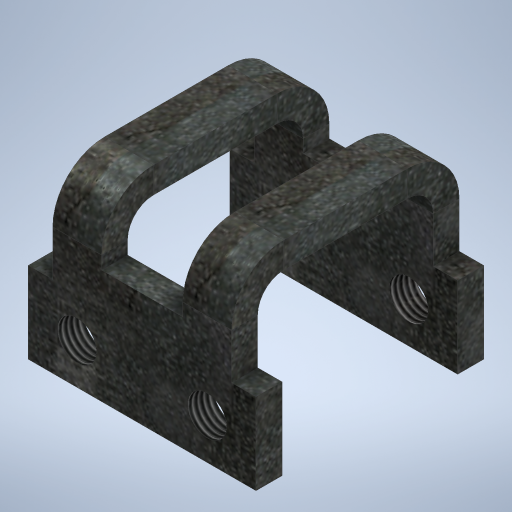
# Autodesk Inventor part: Encaixe Macaco
Saved by Autodesk Inventor 2024 (Build 280153000, 153)
## iProperties
Created: 2024-06-03
Part Number: Encaixe Macaco
Material: Steel ASTM A36
Document SubType Name: Sheet Metal
Designer: Pedro
Density: 7.85 g/cm^3
Sheet Metal Rule: Default_mm
Appearance: Plate
Mass: 418.159 g
Surface Area: 200.819 cm^2
Volume: 53.2687 cm^3
Author: Pedro
Autodesk Inventor part; units mm, degrees
ref_plane "YZ Plane" through (0, 0, 0) normal (1, 0, 0) x (0, 1, 0)
ref_plane "XZ Plane" through (0, 0, 0) normal (0, 1, 0) x (-1, 0, 0)
ref_plane "XY Plane" through (0, 0, 0) normal (0, 0, 1) x (1, 0, 0)
sketch "Sketch1" plane through (0, 0, 0) normal (0, 0, 1) x (1, 0, 0)
  line L0 (2.0005, 12.9652) -> (57.0005, 12.9652)
  line L1 (17.0005, -7.0348) -> (17.0005, 12.9652)
  line L2 (42.0005, 12.9652) -> (42.0005, -7.0348)
  line L3 (42.0005, -7.0348) -> (17.0005, -7.0348)
  line L4 (57.0005, 12.9652) -> (57.0005, -17.0348)
  line L5 (57.0005, -17.0348) -> (64.5005, -17.0348)
  line L6 (64.5005, -17.0348) -> (64.5005, -42.0348)
  line L7 (64.5005, -42.0348) -> (-5.4995, -42.0348)
  line L8 (-5.4995, -42.0348) -> (-5.4995, -17.0348)
  line L9 (-5.4995, -17.0348) -> (2.0005, -17.0348)
  line L10 (2.0005, -17.0348) -> (2.0005, 12.9652)
  point P0 (0, 0)
  point P1 (29.386, -7.0707)
  point P2 (29.5005, -7.0348)
  point P3 (29.5005, 12.9652)
  dimension "d8" = 25
  dimension "d116" = 55
  dimension "d128" = 30
  dimension "d129" = 7.5
  dimension "d130" = 25
  dimension "d131" = 70
  dimension "d132" = 90
  dimension "d133" = 25
  dimension "d134" = 7.5
  dimension "d135" = 27.5
  dimension "d139" = 20
  measures "d8" distance of L1.start L2.end
  measures "d116" distance of L0.start L0.end
  measures "d128" distance of L0.end L4.end
  measures "d129" distance of L4.end L5.end
  measures "d130" distance of L5.end L6.end
  measures "d131" distance of L6.end L7.end
  measures "d132" angle of L6 L7
  measures "d133" distance of L7.end L8.end
  measures "d134" distance of L8.end L9.end
  measures "d135" distance from line of point (29.5, -7.035) L10
  measures "d139" distance of point (29.5, 12.965) point (29.5, -7.035)
extrude "Plate1" add sketch "Sketch1" along normal blind 8 contours L0 L1 L3 L2 L4 L5 L6 L7 L8 L9 L10
sketch "Sketch2" plane through (17.0005, 4.9652, 8) normal (0, 1, 0) x (-1, 0, 0)
  line L0 (15, 0) -> (0, 0)
  line L1 (0, 0) -> (0, -35)
  line L2 (0, -35) -> (15, -35)
  line L3 (15, -35) -> (15, 0)
  constraints: 6 end point, 1 horizontal, 1 perpendicular, 1 vertical
edge flange "Flange1" height 35 angle 90 thickness 8 bend radius 8 thickness toward (0, 1, 0) relief straight relief width 8 relief depth 4 corner gap 8 corner form 0 edges at (9.5005, 12.9652, 0) (49.5005, 12.9652, 0) wall of the first edge with corners at (2.0005, 4.9652, 8) (17.0005, 4.9652, 8) (17.0005, 4.9652, -27) (2.0005, 4.9652, -27)
bend "Bend1"
corner "Corner1"
ref_plane "Work Plane2" through (0, 0, -27) normal (0, 0, 1) x (1, 0, 0)
mirror "Mirror1" about plane through (0, 0, -27) normal (0, 0, 1) of "Plate1"
sketch "Sketch6" plane through (2.0005, 4.9652, -62) normal (0, 1, 0) x (-1, 0, 0)
  line L0 (-15, 0) -> (0, 0)
  line L1 (0, 0) -> (0, 35)
  line L2 (0, 35) -> (-15, 35)
  line L3 (-15, 35) -> (-15, 0)
  constraints: 6 end point, 1 horizontal, 1 perpendicular, 1 vertical
edge flange "Flange4" height 35 angle 90 thickness 8 bend radius 8 thickness toward (0, 1, 0) relief straight relief width 8 relief depth 4 corner gap 8 corner form 0 edges at (9.5005, 12.9652, -54) (49.5005, 12.9652, -54) wall of the first edge with corners at (17.0005, 4.9652, -62) (2.0005, 4.9652, -62) (2.0005, 4.9652, -27) (17.0005, 4.9652, -27)
bend "Bend4"
corner "Corner4"
sketch "Sketch7" plane through (0, 0, 8) normal (0, 0, 1) x (1, 0, 0)
  circle A0 centre (9.5005, -29.5348) radius 6
  circle A1 centre (49.5005, -29.5348) radius 6
  line L0 (-5.4995, -42.0348) -> (-5.4995, -17.0348) projected
  line L1 (64.5005, -42.0348) -> (-5.4995, -42.0348) projected
  point P0 (0, 0)
  point P1 (-5.4995, -29.5348)
  point P2 (29.5005, -42.0348)
  dimension "d55" = 12
  dimension "d56" = 12
  dimension "d57" = 40
  dimension "d136" = 0
  dimension "d137" = 15
  dimension "d138" = 12.5
  constraints: 2 centre point, 2 midpoint
  measures "d55" diameter of A0
  measures "d56" diameter of A1
  measures "d57" distance of A1.centre A0.centre
  measures "d136" vertical distance of A1.centre A0.centre
  measures "d137" distance of point (-5.5, -29.535) A0.centre
  measures "d138" vertical distance of point (29.5, -42.035) A0.centre
extrude "Extrusion1" cut sketch "Sketch7" against normal blind 80
thread "Thread9" size "M12x1.75" class "6H" standard "ANSI Metric M Profile" length 350
thread "Thread10" size "M12x1.75" class "6H" standard "ANSI Metric M Profile" length 350
thread "Thread11" size "M12x1.75" class "6H" standard "ANSI Metric M Profile" length 350
thread "Thread12" size "M12x1.75" class "6H" standard "ANSI Metric M Profile" length 350
equation "\"d12\" = Thickness"
equation "\"d13\" = BendReliefWidth"
equation "\"d14\" = BendReliefDepth"
equation "\"d15\" = MinimumRemnant"
equation "\"d16\" = TransitionRadius"
equation "\"d19\" = BendRadius"
equation "\"d20\" = CornerReliefSize"
equation "\"d21\" = GapSize"
equation "\"d22\" = JacobiRadiusSize"
equation "\"GapSize\" = Thickness"
equation "\"BendRadius\" = Thickness"
equation "\"MinimumRemnant\" = 2 * Thickness"
equation "\"BendReliefDepth\" = 0.5 * Thickness"
equation "\"BendReliefWidth\" = Thickness"
equation "\"CornerReliefSize\" = 4 * Thickness"
equation "\"JacobiRadiusSize\" = BendRadius"
equation "\"TransitionRadius\" = BendRadius"
equation "\"d45\" = BendReliefWidth"
equation "\"d46\" = BendReliefDepth"
equation "\"d47\" = MinimumRemnant"
equation "\"d48\" = TransitionRadius"
equation "\"d51\" = BendRadius"
equation "\"d52\" = CornerReliefSize"
equation "\"d53\" = GapSize"
equation "\"d54\" = JacobiRadiusSize"
equation "\"Thickness\" = 8"
body "Solid1"
